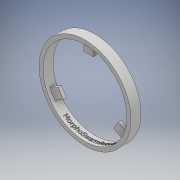
# Autodesk Inventor part: Normal_Ring
Saved by Autodesk Inventor 2018.3 (Build 223284000, 284)
## iProperties
Created: 2021-01-26
Part Number: Normal_Ring
Material: Generic
Document SubType Name: Modeling
Designer: swarmArena
Density: 1 g/cm^3
Appearance: Default
Author: swarmArena
Autodesk Inventor part; units mm, degrees
ref_plane "YZ Plane" through (0, 0, 0) normal (1, 0, 0) x (0, 1, 0)
ref_plane "XZ Plane" through (0, 0, 0) normal (0, 1, 0) x (-1, 0, 0)
ref_plane "XY Plane" through (0, 0, 0) normal (0, 0, 1) x (1, 0, 0)
sketch "Sketch1" plane through (0, 0, 0) normal (0, 1, 0) x (-1, 0, 0)
  line L0 (-23.0349, -9.8524) -> (-17.8647, -6.8674)
  line L1 (-17.8647, -6.8674) -> (-14.8797, -12.0376)
  line L2 (-14.8797, -12.0376) -> (-20.0499, -15.0226)
  line L3 (20.0499, -15.0226) -> (14.8797, -12.0376)
  line L4 (14.8797, -12.0376) -> (17.8647, -6.8674)
  line L5 (17.8647, -6.8674) -> (23.0349, -9.8524)
  line L6 (2.985, 24.875) -> (2.985, 18.905)
  line L7 (2.985, 18.905) -> (-2.985, 18.905)
  line L8 (-2.985, 18.905) -> (-2.985, 24.875)
  circle A0 centre (0, 0) radius 27.5
  arc A1 (23.0349, -9.8524) -> (2.985, 24.875) centre (0, 0) ccw
  arc A2 (-20.0499, -15.0226) -> (20.0499, -15.0226) centre (0, 0) ccw
  arc A3 (-2.985, 24.875) -> (-23.0349, -9.8524) centre (0, 0) ccw
  dimension "d0" = 5.97
  dimension "d1" = 5.97
  dimension "d2" = 55
  constraints: 18 end point, 6 point on circle, 4 centre point, 2 coincident, 1 parallel, 1 perpendicular
  measures "d0" distance of L1.end L2.end
  measures "d1" distance of L1.start L1.end
  measures "d2" diameter of A0
extrude "Extrusion1" add sketch "Sketch1" along normal blind 6
sketch "Sketch2" plane through (0, 0, 0) normal (0, -1, 0) x (1, 0, 0)
  line L0 (-2.985, 18.905) -> (-2.985, 24.875) projected
  line L1 (-2.985, 24.875) -> (-2.985, 18.905)
  line L2 (-2.985, 18.905) -> (2.985, 18.905)
  line L3 (2.985, 18.905) -> (2.985, 24.875) projected
  line L4 (2.985, 18.905) -> (2.985, 24.875)
  arc A0 (2.985, 24.875) -> (-2.985, 24.875) centre (0, 0) ccw
  line L5 (-20.0499, -15.0226) -> (-14.8797, -12.0376)
  line L6 (-14.8797, -12.0376) -> (-17.8647, -6.8674)
  line L7 (-17.8647, -6.8674) -> (-23.0349, -9.8524)
  arc A1 (-23.0349, -9.8524) -> (-20.0499, -15.0226) centre (0, 0) ccw
  line L8 (23.0349, -9.8524) -> (17.8647, -6.8674)
  line L9 (17.8647, -6.8674) -> (14.8797, -12.0376)
  line L10 (14.8797, -12.0376) -> (20.0499, -15.0226)
  arc A2 (20.0499, -15.0226) -> (23.0349, -9.8524) centre (0, 0) ccw
  dimension "d7" = 360
  constraints: 18 end point, 6 point on circle, 3 centre point, 2 collinear, 1 coincident, 1 perpendicular, 28 other
sketch "Sketch3" plane through (0, 6, 0) normal (0, 1, 0) x (1, 0, 0)
  line L0 (-23.0349, 9.8524) -> (-17.8647, 6.8674) projected
  line L1 (-23.0349, 9.8524) -> (-17.8647, 6.8674)
  line L2 (-17.8647, 6.8674) -> (-14.8797, 12.0376) projected
  line L3 (-17.8647, 6.8674) -> (-14.8797, 12.0376)
  arc A0 (20.0499, 15.0226) -> (-20.0499, 15.0226) centre (0, 0) ccw projected
  line L4 (-14.8797, 12.0376) -> (-20.0499, 15.0226)
  arc A1 (-20.0499, 15.0226) -> (-23.0349, 9.8524) centre (0, 0) ccw
  line L5 (2.985, -24.875) -> (2.985, -18.905)
  line L6 (2.985, -18.905) -> (-2.985, -18.905)
  line L7 (-2.985, -18.905) -> (-2.985, -24.875)
  arc A2 (-2.985, -24.875) -> (2.985, -24.875) centre (0, 0) ccw
  line L8 (20.0499, 15.0226) -> (14.8797, 12.0376)
  line L9 (14.8797, 12.0376) -> (17.8647, 6.8674)
  line L10 (17.8647, 6.8674) -> (23.0349, 9.8524)
  arc A3 (23.0349, 9.8524) -> (20.0499, 15.0226) centre (0, 0) ccw
  point P0 (0, 0)
  dimension "d11" = 360
  constraints: 18 end point, 6 point on circle, 3 centre point, 2 collinear, 1 coincident, 1 perpendicular, 28 other
extrude "Extrusion2" cut sketch "Sketch3" against normal blind 2.1
extrude "Extrusion3" cut sketch "Sketch2" against normal blind 2.1
thicken "Thicken1" operation cut thickness 0.15 both sides no extend neighbours no toward (1, 0, 0) faces at (-2.985, 2.7, 20.895) (0.995, 3.3, 18.905) (2.985, 2.7, 20.895)
thicken "Thicken2" operation cut thickness 0.15 both sides no extend neighbours no toward (-0.8660254, 0, -0.5) faces at (-15.8747, 3.3, -10.3142) (-16.6031, 2.7, -13.0326) (-21.3115, 2.7, -8.8574)
thicken "Thicken3" operation cut thickness 0.15 both sides no extend neighbours no toward (0.8660254, 0, -0.5) faces at (16.8697, 3.3, -8.5908) (16.6031, 2.7, -13.0326) (19.5881, 2.7, -7.8624)
thicken "Thicken4" operation add thickness 0.05 both sides no extend neighbours yes toward (-0.6727662, 0, 0.7398551) faces at (-16.8551, 4, 18.5359) (-2.3238, 5.3, 24.9455) (24.2774, 3.3, -6.1872) (20.8187, 5.3, -13.9377) (17.497, 2.7, -17.9313) (-21.8612, 4.6, -12.2377) (2.3238, 1.4, 24.9455) (20.8187, 0.7, -13.9377) (-22.4797, 0.7, -11.0606)
sketch "Sketch5" plane through (0, 0, 0) normal (0, 0, 1) x (1, 0, 0)
  line L0 (-16.2006, 4.4181) -> (17.3036, 4.4181) construction
  line L1 (17.3036, 4.4181) -> (17.3036, -1.7863) construction
  line L2 (17.3036, -1.7863) -> (-16.2006, -1.7863) construction
  line L3 (-16.2006, -1.7863) -> (-16.2006, 4.4181) construction
  line L4 (-13.7656, 1.7649) -> (-14.1031, 1.7649)
  line L5 (-14.1031, 1.7649) -> (-14.1031, 3.9529)
  line L6 (-14.1031, 3.9529) -> (-14.7659, 2.4648)
  line L7 (-14.7659, 2.4648) -> (-14.9717, 2.4648)
  line L8 (-14.9717, 2.4648) -> (-15.6284, 3.9529)
  line L9 (-15.6284, 3.9529) -> (-15.6284, 1.7649)
  line L10 (-15.6284, 1.7649) -> (-15.9433, 1.7649)
  line L11 (-15.9433, 1.7649) -> (-15.9433, 4.3049)
  line L12 (-15.9433, 4.3049) -> (-15.4822, 4.3049)
  line L13 (-15.4822, 4.3049) -> (-14.8482, 2.8908)
  line L14 (-14.8482, 2.8908) -> (-14.2349, 4.3049)
  line L15 (-14.2349, 4.3049) -> (-13.7656, 4.3049)
  line L16 (-13.7656, 4.3049) -> (-13.7656, 1.7649)
  spline S0 degree 2 poles (-11.7093, 2.7179) (-11.7093, 2.2363) (-12.1724, 1.7114) (-12.5594, 1.7114) knots 0 0 0 1 2 2 2
  spline S1 degree 2 poles (-12.5594, 1.7114) (-12.9566, 1.7114) (-13.4115, 2.2528) (-13.4115, 2.7179) knots 0 0 0 1 2 2 2
  spline S2 degree 2 poles (-13.4115, 2.7179) (-13.4115, 3.1955) (-12.9422, 3.7245) (-12.5594, 3.7245) knots 0 0 0 1 2 2 2
  spline S3 degree 2 poles (-12.5594, 3.7245) (-12.1724, 3.7245) (-11.7093, 3.1975) (-11.7093, 2.7179) knots 0 0 0 1 2 2 2
  spline S4 degree 2 poles (-12.0407, 2.7179) (-12.0407, 3.0884) (-12.3103, 3.4487) (-12.5594, 3.4487) knots 0 0 0 1 2 2 2
  spline S5 degree 2 poles (-12.5594, 3.4487) (-12.8084, 3.4487) (-13.0801, 3.0884) (-13.0801, 2.7179) knots 0 0 0 1 2 2 2
  spline S6 degree 2 poles (-13.0801, 2.7179) (-13.0801, 2.3577) (-12.8084, 1.9872) (-12.5594, 1.9872) knots 0 0 0 1 2 2 2
  spline S7 degree 2 poles (-12.5594, 1.9872) (-12.3124, 1.9872) (-12.0407, 2.3516) (-12.0407, 2.7179) knots 0 0 0 1 2 2 2
  line L17 (-10.3693, 3.3272) -> (-10.3857, 3.3272)
  spline S8 degree 2 poles (-10.3857, 3.3272) (-10.4228, 3.3375) (-10.5031, 3.3416) (-10.5587, 3.3416) knots 0 0 0 1 2 2 2
  spline S9 degree 2 poles (-10.5587, 3.3416) (-10.6883, 3.3416) (-10.9436, 3.2284) (-11.0588, 3.1173) knots 0 0 0 1 2 2 2
  line L18 (-11.0588, 3.1173) -> (-11.0588, 1.7649)
  line L19 (-11.0588, 1.7649) -> (-11.3799, 1.7649)
  line L20 (-11.3799, 1.7649) -> (-11.3799, 3.671)
  line L21 (-11.3799, 3.671) -> (-11.0588, 3.671)
  line L22 (-11.0588, 3.671) -> (-11.0588, 3.3869)
  spline S10 degree 2 poles (-11.0588, 3.3869) (-10.8839, 3.5433) (-10.6225, 3.671) (-10.499, 3.671) knots 0 0 0 1 2 2 2
  spline S11 degree 2 poles (-10.499, 3.671) (-10.4496, 3.671) (-10.4002, 3.6668) (-10.3693, 3.6607) knots 0 0 0 1 2 2 2
  line L23 (-10.3693, 3.6607) -> (-10.3693, 3.3272)
  spline S12 degree 2 poles (-8.5229, 2.7694) (-8.5229, 2.2919) (-8.9778, 1.7279) (-9.3257, 1.7279) knots 0 0 0 1 2 2 2
  spline S13 degree 2 poles (-9.3257, 1.7279) (-9.4677, 1.7279) (-9.6859, 1.7937) (-9.7991, 1.8617) knots 0 0 0 1 2 2 2
  line L24 (-9.7991, 1.8617) -> (-9.7991, 1.063)
  line L25 (-9.7991, 1.063) -> (-10.1202, 1.063)
  line L26 (-10.1202, 1.063) -> (-10.1202, 3.671)
  line L27 (-10.1202, 3.671) -> (-9.7991, 3.671)
  line L28 (-9.7991, 3.671) -> (-9.7991, 3.4713)
  spline S14 degree 2 poles (-9.7991, 3.4713) (-9.6797, 3.5804) (-9.3875, 3.7245) (-9.2166, 3.7245) knots 0 0 0 1 2 2 2
  spline S15 degree 2 poles (-9.2166, 3.7245) (-8.8893, 3.7245) (-8.5229, 3.2058) (-8.5229, 2.7694) knots 0 0 0 1 2 2 2
  spline S16 degree 2 poles (-8.8543, 2.7323) (-8.8543, 3.0596) (-9.0622, 3.4198) (-9.2948, 3.4198) knots 0 0 0 1 2 2 2
  spline S17 degree 2 poles (-9.2948, 3.4198) (-9.4307, 3.4198) (-9.6859, 3.2984) (-9.7991, 3.2037) knots 0 0 0 1 2 2 2
  line L29 (-9.7991, 3.2037) -> (-9.7991, 2.121)
  spline S18 degree 2 poles (-9.7991, 2.121) (-9.6736, 2.0613) (-9.4945, 2.016) (-9.3792, 2.016) knots 0 0 0 1 2 2 2
  spline S19 degree 2 poles (-9.3792, 2.016) (-9.1302, 2.016) (-8.8543, 2.3824) (-8.8543, 2.7323) knots 0 0 0 1 2 2 2
  line L30 (-6.6931, 1.7649) -> (-7.0142, 1.7649)
  line L31 (-7.0142, 1.7649) -> (-7.0142, 2.8517)
  spline S20 degree 2 poles (-7.0142, 2.8517) (-7.0142, 2.9835) (-7.0389, 3.2099) (-7.0759, 3.2778) knots 0 0 0 1 2 2 2
  spline S21 degree 2 poles (-7.0759, 3.2778) (-7.115, 3.3499) (-7.255, 3.4198) (-7.3744, 3.4198) knots 0 0 0 1 2 2 2
  spline S22 degree 2 poles (-7.3744, 3.4198) (-7.4938, 3.4198) (-7.7469, 3.2922) (-7.8684, 3.1893) knots 0 0 0 1 2 2 2
  line L32 (-7.8684, 3.1893) -> (-7.8684, 1.7649)
  line L33 (-7.8684, 1.7649) -> (-8.1895, 1.7649)
  line L34 (-8.1895, 1.7649) -> (-8.1895, 4.4181)
  line L35 (-8.1895, 4.4181) -> (-7.8684, 4.4181)
  line L36 (-7.8684, 4.4181) -> (-7.8684, 3.4589)
  spline S23 degree 2 poles (-7.8684, 3.4589) (-7.7243, 3.5886) (-7.4464, 3.7245) (-7.29, 3.7245) knots 0 0 0 1 2 2 2
  spline S24 degree 2 poles (-7.29, 3.7245) (-7.0101, 3.7245) (-6.6931, 3.354) (-6.6931, 3.002) knots 0 0 0 1 2 2 2
  line L37 (-6.6931, 3.002) -> (-6.6931, 1.7649)
  spline S25 degree 2 poles (-4.6759, 2.7179) (-4.6759, 2.2363) (-5.139, 1.7114) (-5.526, 1.7114) knots 0 0 0 1 2 2 2
  spline S26 degree 2 poles (-5.526, 1.7114) (-5.9233, 1.7114) (-6.3781, 2.2528) (-6.3781, 2.7179) knots 0 0 0 1 2 2 2
  spline S27 degree 2 poles (-6.3781, 2.7179) (-6.3781, 3.1955) (-5.9088, 3.7245) (-5.526, 3.7245) knots 0 0 0 1 2 2 2
  spline S28 degree 2 poles (-5.526, 3.7245) (-5.139, 3.7245) (-4.6759, 3.1975) (-4.6759, 2.7179) knots 0 0 0 1 2 2 2
  spline S29 degree 2 poles (-5.0073, 2.7179) (-5.0073, 3.0884) (-5.2769, 3.4487) (-5.526, 3.4487) knots 0 0 0 1 2 2 2
  spline S30 degree 2 poles (-5.526, 3.4487) (-5.7751, 3.4487) (-6.0468, 3.0884) (-6.0468, 2.7179) knots 0 0 0 1 2 2 2
  spline S31 degree 2 poles (-6.0468, 2.7179) (-6.0468, 2.3577) (-5.7751, 1.9872) (-5.526, 1.9872) knots 0 0 0 1 2 2 2
  spline S32 degree 2 poles (-5.526, 1.9872) (-5.279, 1.9872) (-5.0073, 2.3516) (-5.0073, 2.7179) knots 0 0 0 1 2 2 2
  spline S33 degree 2 poles (-3.6138, 1.7196) (-3.8896, 1.7196) (-4.2766, 1.8349) (-4.4474, 1.9172) knots 0 0 0 1 2 2 2
  line L38 (-4.4474, 1.9172) -> (-4.4474, 2.3413)
  line L39 (-4.4474, 2.3413) -> (-4.4227, 2.3413)
  spline S34 degree 2 poles (-4.4227, 2.3413) (-4.256, 2.1848) (-3.834, 2.0119) (-3.6385, 2.0119) knots 0 0 0 1 2 2 2
  spline S35 degree 2 poles (-3.6385, 2.0119) (-3.3586, 2.0119) (-3.0724, 2.2445) (-3.0724, 2.4359) knots 0 0 0 1 2 2 2
  spline S36 degree 2 poles (-3.0724, 2.4359) (-3.0724, 2.5883) (-3.2227, 2.7776) (-3.3853, 2.825) knots 0 0 0 1 2 2 2
  spline S37 degree 2 poles (-3.3853, 2.825) (-3.5026, 2.8579) (-3.6982, 2.9032) (-3.8443, 2.9402) knots 0 0 0 1 2 2 2
  spline S38 degree 2 poles (-3.8443, 2.9402) (-3.9761, 2.9752) (-4.184, 3.0802) (-4.2642, 3.1646) knots 0 0 0 1 2 2 2
  spline S39 degree 2 poles (-4.2642, 3.1646) (-4.3424, 3.249) (-4.4289, 3.4754) (-4.4289, 3.6236) knots 0 0 0 1 2 2 2
  spline S40 degree 2 poles (-4.4289, 3.6236) (-4.4289, 3.9324) (-3.9472, 4.3502) (-3.5747, 4.3502) knots 0 0 0 1 2 2 2
  spline S41 degree 2 poles (-3.5747, 4.3502) (-3.3606, 4.3502) (-2.9819, 4.2658) (-2.8193, 4.1855) knots 0 0 0 1 2 2 2
  line L40 (-2.8193, 4.1855) -> (-2.8193, 3.7821)
  line L41 (-2.8193, 3.7821) -> (-2.844, 3.7821)
  spline S42 degree 2 poles (-2.844, 3.7821) (-2.9654, 3.8933) (-3.3441, 4.0579) (-3.552, 4.0579) knots 0 0 0 1 2 2 2
  spline S43 degree 2 poles (-3.552, 4.0579) (-3.7867, 4.0579) (-4.0769, 3.8377) (-4.0769, 3.6586) knots 0 0 0 1 2 2 2
  spline S44 degree 2 poles (-4.0769, 3.6586) (-4.0769, 3.4981) (-3.9061, 3.3066) (-3.7455, 3.2634) knots 0 0 0 1 2 2 2
  spline S45 degree 2 poles (-3.7455, 3.2634) (-3.6385, 3.2346) (-3.3277, 3.1605) (-3.2248, 3.1296) knots 0 0 0 1 2 2 2
  spline S46 degree 2 poles (-3.2248, 3.1296) (-2.9634, 3.0493) (-2.7205, 2.7262) (-2.7205, 2.4895) knots 0 0 0 1 2 2 2
  spline S47 degree 2 poles (-2.7205, 2.4895) (-2.7205, 2.3392) (-2.8419, 2.051) (-2.951, 1.9502) knots 0 0 0 1 2 2 2
  spline S48 degree 2 poles (-2.951, 1.9502) (-3.0724, 1.839) (-3.3812, 1.7196) (-3.6138, 1.7196) knots 0 0 0 1 2 2 2
  line L42 (-0.092, 3.671) -> (-0.5757, 1.7649)
  line L43 (-0.5757, 1.7649) -> (-0.8721, 1.7649)
  line L44 (-0.8721, 1.7649) -> (-1.3373, 3.2346)
  line L45 (-1.3373, 3.2346) -> (-1.8004, 1.7649)
  line L46 (-1.8004, 1.7649) -> (-2.0947, 1.7649)
  line L47 (-2.0947, 1.7649) -> (-2.5826, 3.671)
  line L48 (-2.5826, 3.671) -> (-2.2491, 3.671)
  line L49 (-2.2491, 3.671) -> (-1.9115, 2.1951)
  line L50 (-1.9115, 2.1951) -> (-1.4608, 3.671)
  line L51 (-1.4608, 3.671) -> (-1.1952, 3.671)
  line L52 (-1.1952, 3.671) -> (-0.7321, 2.1951)
  line L53 (-0.7321, 2.1951) -> (-0.4151, 3.671)
  line L54 (-0.4151, 3.671) -> (-0.092, 3.671)
  spline S49 degree 2 poles (1.2521, 1.9666) (1.213, 1.9378) (1.0813, 1.8349) (1.0196, 1.804) knots 0 0 0 1 2 2 2
  spline S50 degree 2 poles (1.0196, 1.804) (0.9352, 1.7588) (0.7767, 1.7114) (0.6326, 1.7114) knots 0 0 0 1 2 2 2
  spline S51 degree 2 poles (0.6326, 1.7114) (0.5153, 1.7114) (0.3032, 1.7999) (0.223, 1.8802) knots 0 0 0 1 2 2 2
  spline S52 degree 2 poles (0.223, 1.8802) (0.1468, 1.9584) (0.0542, 2.1889) (0.0542, 2.3166) knots 0 0 0 1 2 2 2
  spline S53 degree 2 poles (0.0542, 2.3166) (0.0542, 2.5142) (0.2209, 2.7941) (0.402, 2.8744) knots 0 0 0 1 2 2 2
  spline S54 degree 2 poles (0.402, 2.8744) (0.5626, 2.9485) (0.999, 3.0041) (1.2521, 3.0185) knots 0 0 0 1 2 2 2
  line L55 (1.2521, 3.0185) -> (1.2521, 3.0802)
  spline S55 degree 2 poles (1.2521, 3.0802) (1.2521, 3.1914) (1.1842, 3.3293) (1.1225, 3.3684) knots 0 0 0 1 2 2 2
  spline S56 degree 2 poles (1.1225, 3.3684) (1.0607, 3.4075) (0.8837, 3.4322) (0.789, 3.4322) knots 0 0 0 1 2 2 2
  spline S57 degree 2 poles (0.789, 3.4322) (0.6779, 3.4322) (0.3773, 3.3663) (0.2271, 3.3025) knots 0 0 0 1 2 2 2
  line L56 (0.2271, 3.3025) -> (0.2086, 3.3025)
  line L57 (0.2086, 3.3025) -> (0.2086, 3.6298)
  spline S58 degree 2 poles (0.2086, 3.6298) (0.2971, 3.6545) (0.6285, 3.7162) (0.7911, 3.7162) knots 0 0 0 1 2 2 2
  spline S59 degree 2 poles (0.7911, 3.7162) (0.9887, 3.7162) (1.2583, 3.6545) (1.3654, 3.5742) knots 0 0 0 1 2 2 2
  spline S60 degree 2 poles (1.3654, 3.5742) (1.4703, 3.496) (1.5732, 3.2469) (1.5732, 3.0679) knots 0 0 0 1 2 2 2
  line L58 (1.5732, 3.0679) -> (1.5732, 1.7649)
  line L59 (1.5732, 1.7649) -> (1.2521, 1.7649)
  line L60 (1.2521, 1.7649) -> (1.2521, 1.9666)
  line L61 (1.2521, 2.2342) -> (1.2521, 2.7632)
  spline S61 degree 2 poles (1.2521, 2.7632) (1.1369, 2.7529) (0.789, 2.7179) (0.6799, 2.685) knots 0 0 0 1 2 2 2
  spline S62 degree 2 poles (0.6799, 2.685) (0.5523, 2.6459) (0.3856, 2.4833) (0.3856, 2.3392) knots 0 0 0 1 2 2 2
  spline S63 degree 2 poles (0.3856, 2.3392) (0.3856, 2.1745) (0.5708, 2.0078) (0.7478, 2.0078) knots 0 0 0 1 2 2 2
  spline S64 degree 2 poles (0.7478, 2.0078) (0.8981, 2.0078) (1.1451, 2.1375) (1.2521, 2.2342) knots 0 0 0 1 2 2 2
  line L62 (3.0347, 3.3272) -> (3.0182, 3.3272)
  spline S65 degree 2 poles (3.0182, 3.3272) (2.9812, 3.3375) (2.9009, 3.3416) (2.8453, 3.3416) knots 0 0 0 1 2 2 2
  spline S66 degree 2 poles (2.8453, 3.3416) (2.7156, 3.3416) (2.4604, 3.2284) (2.3451, 3.1173) knots 0 0 0 1 2 2 2
  line L63 (2.3451, 3.1173) -> (2.3451, 1.7649)
  line L64 (2.3451, 1.7649) -> (2.024, 1.7649)
  line L65 (2.024, 1.7649) -> (2.024, 3.671)
  line L66 (2.024, 3.671) -> (2.3451, 3.671)
  line L67 (2.3451, 3.671) -> (2.3451, 3.3869)
  spline S67 degree 2 poles (2.3451, 3.3869) (2.5201, 3.5433) (2.7815, 3.671) (2.905, 3.671) knots 0 0 0 1 2 2 2
  spline S68 degree 2 poles (2.905, 3.671) (2.9544, 3.671) (3.0038, 3.6668) (3.0347, 3.6607) knots 0 0 0 1 2 2 2
  line L68 (3.0347, 3.6607) -> (3.0347, 3.3272)
  line L69 (5.445, 1.7649) -> (5.445, 2.8682)
  spline S69 degree 2 poles (5.445, 2.8682) (5.445, 2.9999) (5.4244, 3.2243) (5.3915, 3.286) knots 0 0 0 1 2 2 2
  spline S70 degree 2 poles (5.3915, 3.286) (5.3585, 3.354) (5.233, 3.4198) (5.1239, 3.4198) knots 0 0 0 1 2 2 2
  spline S71 degree 2 poles (5.1239, 3.4198) (5.0251, 3.4198) (4.7987, 3.2984) (4.6793, 3.1831) knots 0 0 0 1 2 2 2
  spline S72 degree 2 poles (4.6793, 3.1831) (4.6813, 3.1543) (4.6855, 3.074) (4.6855, 3.0205) knots 0 0 0 1 2 2 2
  line L70 (4.6855, 3.0205) -> (4.6855, 1.7649)
  line L71 (4.6855, 1.7649) -> (4.3644, 1.7649)
  line L72 (4.3644, 1.7649) -> (4.3644, 2.8682)
  spline S73 degree 2 poles (4.3644, 2.8682) (4.3644, 2.9999) (4.3438, 3.2243) (4.3108, 3.286) knots 0 0 0 1 2 2 2
  spline S74 degree 2 poles (4.3108, 3.286) (4.2779, 3.354) (4.1524, 3.4198) (4.0433, 3.4198) knots 0 0 0 1 2 2 2
  spline S75 degree 2 poles (4.0433, 3.4198) (3.9403, 3.4198) (3.7119, 3.2902) (3.6048, 3.1893) knots 0 0 0 1 2 2 2
  line L73 (3.6048, 3.1893) -> (3.6048, 1.7649)
  line L74 (3.6048, 1.7649) -> (3.2837, 1.7649)
  line L75 (3.2837, 1.7649) -> (3.2837, 3.671)
  line L76 (3.2837, 3.671) -> (3.6048, 3.671)
  line L77 (3.6048, 3.671) -> (3.6048, 3.461)
  spline S76 degree 2 poles (3.6048, 3.461) (3.7304, 3.5866) (3.9774, 3.7245) (4.1256, 3.7245) knots 0 0 0 1 2 2 2
  spline S77 degree 2 poles (4.1256, 3.7245) (4.2944, 3.7245) (4.5558, 3.5701) (4.6237, 3.3951) knots 0 0 0 1 2 2 2
  spline S78 degree 2 poles (4.6237, 3.3951) (4.7699, 3.5577) (5.0457, 3.7245) (5.2062, 3.7245) knots 0 0 0 1 2 2 2
  spline S79 degree 2 poles (5.2062, 3.7245) (5.3297, 3.7245) (5.5314, 3.6483) (5.6055, 3.5619) knots 0 0 0 1 2 2 2
  spline S80 degree 2 poles (5.6055, 3.5619) (5.6817, 3.4754) (5.7661, 3.2161) (5.7661, 3.0205) knots 0 0 0 1 2 2 2
  line L78 (5.7661, 3.0205) -> (5.7661, 1.7649)
  line L79 (5.7661, 1.7649) -> (5.445, 1.7649)
  line L80 (8.2073, 1.7649) -> (7.7689, 1.7649)
  line L81 (7.7689, 1.7649) -> (6.9661, 2.7756)
  line L82 (6.9661, 2.7756) -> (6.5791, 2.7756)
  line L83 (6.5791, 2.7756) -> (6.5791, 1.7649)
  line L84 (6.5791, 1.7649) -> (6.2416, 1.7649)
  line L85 (6.2416, 1.7649) -> (6.2416, 4.3049)
  line L86 (6.2416, 4.3049) -> (6.8961, 4.3049)
  spline S81 degree 2 poles (6.8961, 4.3049) (7.1143, 4.3049) (7.4087, 4.2576) (7.5425, 4.1711) knots 0 0 0 1 2 2 2
  spline S82 degree 2 poles (7.5425, 4.1711) (7.6762, 4.0847) (7.8306, 3.815) (7.8306, 3.6154) knots 0 0 0 1 2 2 2
  spline S83 degree 2 poles (7.8306, 3.6154) (7.8306, 3.3375) (7.5466, 2.9608) (7.3037, 2.8703) knots 0 0 0 1 2 2 2
  line L87 (7.3037, 2.8703) -> (8.2073, 1.7649)
  spline S84 degree 2 poles (7.4786, 3.5886) (7.4786, 3.6998) (7.4004, 3.8706) (7.3181, 3.9262) knots 0 0 0 1 2 2 2
  spline S85 degree 2 poles (7.3181, 3.9262) (7.246, 3.9735) (7.0546, 4.0126) (6.9147, 4.0126) knots 0 0 0 1 2 2 2
  line L88 (6.9147, 4.0126) -> (6.5791, 4.0126)
  line L89 (6.5791, 4.0126) -> (6.5791, 3.0576)
  line L90 (6.5791, 3.0576) -> (6.8755, 3.0576)
  spline S86 degree 2 poles (6.8755, 3.0576) (7.0217, 3.0576) (7.2543, 3.109) (7.3346, 3.1893) knots 0 0 0 1 2 2 2
  spline S87 degree 2 poles (7.3346, 3.1893) (7.4087, 3.2593) (7.4786, 3.4569) (7.4786, 3.5886) knots 0 0 0 1 2 2 2
  spline S88 degree 2 poles (9.9507, 2.7179) (9.9507, 2.2363) (9.4876, 1.7114) (9.1006, 1.7114) knots 0 0 0 1 2 2 2
  spline S89 degree 2 poles (9.1006, 1.7114) (8.7034, 1.7114) (8.2485, 2.2528) (8.2485, 2.7179) knots 0 0 0 1 2 2 2
  spline S90 degree 2 poles (8.2485, 2.7179) (8.2485, 3.1955) (8.7178, 3.7245) (9.1006, 3.7245) knots 0 0 0 1 2 2 2
  spline S91 degree 2 poles (9.1006, 3.7245) (9.4876, 3.7245) (9.9507, 3.1975) (9.9507, 2.7179) knots 0 0 0 1 2 2 2
  spline S92 degree 2 poles (9.6193, 2.7179) (9.6193, 3.0884) (9.3497, 3.4487) (9.1006, 3.4487) knots 0 0 0 1 2 2 2
  spline S93 degree 2 poles (9.1006, 3.4487) (8.8516, 3.4487) (8.5799, 3.0884) (8.5799, 2.7179) knots 0 0 0 1 2 2 2
  spline S94 degree 2 poles (8.5799, 2.7179) (8.5799, 2.3577) (8.8516, 1.9872) (9.1006, 1.9872) knots 0 0 0 1 2 2 2
  spline S95 degree 2 poles (9.1006, 1.9872) (9.3476, 1.9872) (9.6193, 2.3516) (9.6193, 2.7179) knots 0 0 0 1 2 2 2
  spline S96 degree 2 poles (11.8773, 2.7488) (11.8773, 2.2816) (11.4245, 1.7114) (11.0828, 1.7114) knots 0 0 0 1 2 2 2
  spline S97 degree 2 poles (11.0828, 1.7114) (10.9284, 1.7114) (10.7082, 1.7876) (10.6012, 1.8534) knots 0 0 0 1 2 2 2
  line L91 (10.6012, 1.8534) -> (10.5806, 1.7649)
  line L92 (10.5806, 1.7649) -> (10.2801, 1.7649)
  line L93 (10.2801, 1.7649) -> (10.2801, 4.4181)
  line L94 (10.2801, 4.4181) -> (10.6012, 4.4181)
  line L95 (10.6012, 4.4181) -> (10.6012, 3.4713)
  spline S98 degree 2 poles (10.6012, 3.4713) (10.7226, 3.5804) (11.0046, 3.7245) (11.1837, 3.7245) knots 0 0 0 1 2 2 2
  spline S99 degree 2 poles (11.1837, 3.7245) (11.5068, 3.7245) (11.8773, 3.2078) (11.8773, 2.7488) knots 0 0 0 1 2 2 2
  spline S100 degree 2 poles (11.5459, 2.7241) (11.5459, 3.0658) (11.338, 3.4198) (11.1075, 3.4198) knots 0 0 0 1 2 2 2
  spline S101 degree 2 poles (11.1075, 3.4198) (10.9778, 3.4198) (10.7102, 3.2963) (10.6012, 3.2017) knots 0 0 0 1 2 2 2
  line L96 (10.6012, 3.2017) -> (10.6012, 2.1087)
  spline S102 degree 2 poles (10.6012, 2.1087) (10.7226, 2.049) (10.9099, 1.9996) (11.0211, 1.9996) knots 0 0 0 1 2 2 2
  spline S103 degree 2 poles (11.0211, 1.9996) (11.266, 1.9996) (11.5459, 2.3474) (11.5459, 2.7241) knots 0 0 0 1 2 2 2
  spline S104 degree 2 poles (13.7772, 2.7179) (13.7772, 2.2363) (13.3141, 1.7114) (12.9271, 1.7114) knots 0 0 0 1 2 2 2
  spline S105 degree 2 poles (12.9271, 1.7114) (12.5298, 1.7114) (12.0749, 2.2528) (12.0749, 2.7179) knots 0 0 0 1 2 2 2
  spline S106 degree 2 poles (12.0749, 2.7179) (12.0749, 3.1955) (12.5442, 3.7245) (12.9271, 3.7245) knots 0 0 0 1 2 2 2
  spline S107 degree 2 poles (12.9271, 3.7245) (13.3141, 3.7245) (13.7772, 3.1975) (13.7772, 2.7179) knots 0 0 0 1 2 2 2
  spline S108 degree 2 poles (13.4458, 2.7179) (13.4458, 3.0884) (13.1761, 3.4487) (12.9271, 3.4487) knots 0 0 0 1 2 2 2
  spline S109 degree 2 poles (12.9271, 3.4487) (12.678, 3.4487) (12.4063, 3.0884) (12.4063, 2.7179) knots 0 0 0 1 2 2 2
  spline S110 degree 2 poles (12.4063, 2.7179) (12.4063, 2.3577) (12.678, 1.9872) (12.9271, 1.9872) knots 0 0 0 1 2 2 2
  spline S111 degree 2 poles (12.9271, 1.9872) (13.1741, 1.9872) (13.4458, 2.3516) (13.4458, 2.7179) knots 0 0 0 1 2 2 2
  spline S112 degree 2 poles (14.6829, 1.7279) (14.4214, 1.7279) (14.1271, 2.0263) (14.1271, 2.3495) knots 0 0 0 1 2 2 2
  line L97 (14.1271, 2.3495) -> (14.1271, 3.4054)
  line L98 (14.1271, 3.4054) -> (13.911, 3.4054)
  line L99 (13.911, 3.4054) -> (13.911, 3.671)
  line L100 (13.911, 3.671) -> (14.1271, 3.671)
  line L101 (14.1271, 3.671) -> (14.1271, 4.2185)
  line L102 (14.1271, 4.2185) -> (14.4482, 4.2185)
  line L103 (14.4482, 4.2185) -> (14.4482, 3.671)
  line L104 (14.4482, 3.671) -> (15.039, 3.671)
  line L105 (15.039, 3.671) -> (15.039, 3.4054)
  line L106 (15.039, 3.4054) -> (14.4482, 3.4054)
  line L107 (14.4482, 3.4054) -> (14.4482, 2.4977)
  spline S113 degree 2 poles (14.4482, 2.4977) (14.4482, 2.3536) (14.4585, 2.1951) (14.4935, 2.1272) knots 0 0 0 1 2 2 2
  spline S114 degree 2 poles (14.4935, 2.1272) (14.5223, 2.0675) (14.652, 2.0078) (14.7631, 2.0078) knots 0 0 0 1 2 2 2
  spline S115 degree 2 poles (14.7631, 2.0078) (14.8413, 2.0078) (14.9875, 2.0552) (15.0204, 2.0696) knots 0 0 0 1 2 2 2
  line L108 (15.0204, 2.0696) -> (15.039, 2.0696)
  line L109 (15.039, 2.0696) -> (15.039, 1.7814)
  spline S116 degree 2 poles (15.039, 1.7814) (14.9484, 1.7567) (14.7631, 1.7279) (14.6829, 1.7279) knots 0 0 0 1 2 2 2
  line L110 (15.6029, 1.7649) -> (15.2818, 1.7649)
  line L111 (15.2818, 1.7649) -> (15.2818, 3.671)
  line L112 (15.2818, 3.671) -> (15.6029, 3.671)
  line L113 (15.6029, 3.671) -> (15.6029, 1.7649)
  line L114 (15.6256, 3.9879) -> (15.2613, 3.9879)
  line L115 (15.2613, 3.9879) -> (15.2613, 4.3214)
  line L116 (15.2613, 4.3214) -> (15.6256, 4.3214)
  line L117 (15.6256, 4.3214) -> (15.6256, 3.9879)
  spline S117 degree 2 poles (16.8318, 1.7217) (16.6342, 1.7217) (16.3069, 1.8431) (16.1896, 1.9666) knots 0 0 0 1 2 2 2
  spline S118 degree 2 poles (16.1896, 1.9666) (16.0722, 2.0881) (15.9426, 2.4627) (15.9426, 2.7138) knots 0 0 0 1 2 2 2
  spline S119 degree 2 poles (15.9426, 2.7138) (15.9426, 2.9649) (16.0764, 3.3313) (16.1896, 3.4548) knots 0 0 0 1 2 2 2
  spline S120 degree 2 poles (16.1896, 3.4548) (16.3028, 3.5804) (16.6383, 3.7142) (16.8318, 3.7142) knots 0 0 0 1 2 2 2
  spline S121 degree 2 poles (16.8318, 3.7142) (16.9882, 3.7142) (17.2805, 3.6257) (17.3937, 3.568) knots 0 0 0 1 2 2 2
  line L118 (17.3937, 3.568) -> (17.3937, 3.2078)
  line L119 (17.3937, 3.2078) -> (17.3752, 3.2078)
  spline S122 degree 2 poles (17.3752, 3.2078) (17.3402, 3.2366) (17.2331, 3.3107) (17.157, 3.3499) knots 0 0 0 1 2 2 2
  spline S123 degree 2 poles (17.157, 3.3499) (17.0891, 3.3828) (16.9079, 3.4342) (16.8256, 3.4342) knots 0 0 0 1 2 2 2
  spline S124 degree 2 poles (16.8256, 3.4342) (16.5765, 3.4342) (16.274, 3.0576) (16.274, 2.7138) knots 0 0 0 1 2 2 2
  spline S125 degree 2 poles (16.274, 2.7138) (16.274, 2.3783) (16.5662, 2.0016) (16.8256, 2.0016) knots 0 0 0 1 2 2 2
  spline S126 degree 2 poles (16.8256, 2.0016) (16.982, 2.0016) (17.2661, 2.1313) (17.3752, 2.2322) knots 0 0 0 1 2 2 2
  line L120 (17.3752, 2.2322) -> (17.3937, 2.2322)
  line L121 (17.3937, 2.2322) -> (17.3937, 1.872)
  spline S127 degree 2 poles (17.3937, 1.872) (17.3464, 1.8493) (17.2023, 1.7855) (17.1446, 1.7711) knots 0 0 0 1 2 2 2
  spline S128 degree 2 poles (17.1446, 1.7711) (17.0623, 1.7464) (16.9326, 1.7217) (16.8318, 1.7217) knots 0 0 0 1 2 2 2
  spline S129 degree 2 poles (18.2006, 1.7196) (18.0091, 1.7196) (17.6778, 1.8226) (17.5687, 1.8802) knots 0 0 0 1 2 2 2
  line L122 (17.5687, 1.8802) -> (17.5687, 2.2404)
  line L123 (17.5687, 2.2404) -> (17.5851, 2.2404)
  spline S130 degree 2 poles (17.5851, 2.2404) (17.6263, 2.2075) (17.7374, 2.1293) (17.8301, 2.086) knots 0 0 0 1 2 2 2
  spline S131 degree 2 poles (17.8301, 2.086) (17.9103, 2.0469) (18.1079, 1.9893) (18.2129, 1.9893) knots 0 0 0 1 2 2 2
  spline S132 degree 2 poles (18.2129, 1.9893) (18.2891, 1.9893) (18.464, 2.0243) (18.5052, 2.0531) knots 0 0 0 1 2 2 2
  spline S133 degree 2 poles (18.5052, 2.0531) (18.5649, 2.0922) (18.6184, 2.1807) (18.6184, 2.2713) knots 0 0 0 1 2 2 2
  spline S134 degree 2 poles (18.6184, 2.2713) (18.6184, 2.3845) (18.4949, 2.5018) (18.3364, 2.5409) knots 0 0 0 1 2 2 2
  spline S135 degree 2 poles (18.3364, 2.5409) (18.2747, 2.5553) (18.0771, 2.5965) (17.9927, 2.6191) knots 0 0 0 1 2 2 2
  spline S136 degree 2 poles (17.9927, 2.6191) (17.7745, 2.6829) (17.5769, 2.9464) (17.5769, 3.1337) knots 0 0 0 1 2 2 2
  spline S137 degree 2 poles (17.5769, 3.1337) (17.5769, 3.3931) (17.9659, 3.7162) (18.287, 3.7162) knots 0 0 0 1 2 2 2
  spline S138 degree 2 poles (18.287, 3.7162) (18.4455, 3.7162) (18.7666, 3.638) (18.8757, 3.5783) knots 0 0 0 1 2 2 2
  line L124 (18.8757, 3.5783) -> (18.8757, 3.2346)
  line L125 (18.8757, 3.2346) -> (18.8592, 3.2346)
  spline S139 degree 2 poles (18.8592, 3.2346) (18.7357, 3.3334) (18.4352, 3.4466) (18.2808, 3.4466) knots 0 0 0 1 2 2 2
  spline S140 degree 2 poles (18.2808, 3.4466) (18.1224, 3.4466) (17.9042, 3.3128) (17.9042, 3.179) knots 0 0 0 1 2 2 2
  spline S141 degree 2 poles (17.9042, 3.179) (17.9042, 3.0576) (18.0338, 2.9402) (18.1779, 2.9032) knots 0 0 0 1 2 2 2
  spline S142 degree 2 poles (18.1779, 2.9032) (18.2479, 2.8847) (18.4249, 2.8476) (18.5217, 2.825) knots 0 0 0 1 2 2 2
  spline S143 degree 2 poles (18.5217, 2.825) (18.7316, 2.7715) (18.9457, 2.5265) (18.9457, 2.3145) knots 0 0 0 1 2 2 2
  spline S144 degree 2 poles (18.9457, 2.3145) (18.9457, 2.191) (18.849, 1.9728) (18.7543, 1.8925) knots 0 0 0 1 2 2 2
  spline S145 degree 2 poles (18.7543, 1.8925) (18.6534, 1.8082) (18.3961, 1.7196) (18.2006, 1.7196) knots 0 0 0 1 2 2 2
  point P0 (0, 0)
  constraints: 2 other
emboss "Emboss1" sketch "Sketch5" operation cut depth 0.5 direction (0, 0, 1) wrap yes faces at (-12.1672, 2, 21.9578) (0.3331, 4.6, 25.1012) (15.4038, 4, 19.8219) (21.5718, 4.6, -12.8391) (9.4644, 4, -23.251) (-21.9049, 4.6, -12.2621) (0.3331, 1.4, 25.1012) (21.5718, 1.4, -12.8391) (-21.9049, 1.4, -12.2621)
body "Solid1"
